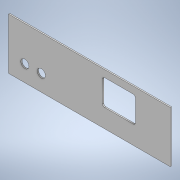
# Autodesk Inventor part: BackPanel
Saved by Autodesk Inventor 2021.4 (Build 254397000, 397)
## iProperties
Created: 2022-05-18
Part Number: BackPanel
Material: Generic
Document SubType Name: Modeling
Designer: LaborAdmin
Density: 1 g/cm^3
Appearance: Default
Author: LaborAdmin
Autodesk Inventor part; units mm, degrees
ref_plane "YZ Plane" through (0, 0, 0) normal (1, 0, 0) x (0, 1, 0)
ref_plane "XZ Plane" through (0, 0, 0) normal (0, 1, 0) x (-1, 0, 0)
ref_plane "XY Plane" through (0, 0, 0) normal (0, 0, 1) x (1, 0, 0)
sketch "Sketch1" plane through (0, 0, 0) normal (0, 0, 1) x (1, 0, 0)
  line L0 (-197, 62.5) -> (197, 62.5)
  line L1 (197, 62.5) -> (197, -62.5)
  line L2 (197, -62.5) -> (-197, -62.5)
  line L3 (-197, -62.5) -> (-197, 62.5)
  line L4 (-197, 62.5) -> (197, -62.5) construction
  line L5 (197, 62.5) -> (-197, -62.5) construction
  point P0 (0, 0)
  dimension "d0" = 394
  dimension "d1" = 125
  constraints: 12 end point, 2 midpoint, 2 parallel, 1 horizontal, 1 perpendicular
  measures "d0" distance of L1.end L2.end
  measures "d1" distance of L0.end L1.end
extrude "Extrusion1" add sketch "Sketch1" against normal blind 3
sketch "Sketch2" plane through (0, 0, 0) normal (0, 0, 1) x (1, 0, 0)
  circle A0 centre (-157, -22.5) radius 10
  circle A1 centre (-117, -22.5) radius 10
  line L0 (-197, -62.5) -> (197, -62.5) projected
  line L1 (-197, 62.5) -> (-197, -62.5) projected
  line L2 (37, 45.5) -> (107, 45.5)
  line L3 (112, 40.5) -> (112, -12.5)
  line L4 (107, -17.5) -> (37, -17.5)
  line L5 (32, -12.5) -> (32, 40.5)
  line L6 (197, 62.5) -> (-197, 62.5) projected
  line L7 (197, -62.5) -> (197, 62.5) projected
  arc A2 (37, 45.5) -> (32, 40.5) centre (37, 40.5) ccw
  arc A3 (112, 40.5) -> (107, 45.5) centre (107, 40.5) ccw
  arc A4 (107, -17.5) -> (112, -12.5) centre (107, -12.5) ccw
  arc A5 (32, -12.5) -> (37, -17.5) centre (37, -12.5) ccw
  point P0 (0, 0)
  point P1 (32, 45.5)
  point P2 (112, -17.5)
  point P3 (112, 45.5)
  point P4 (32, -17.5)
  dimension "d4" = 20
  dimension "USB" = 20
  dimension "d6" = 40
  dimension "d7" = 40
  dimension "d8" = 40
  dimension "d9" = 40
  dimension "d10" = 63
  dimension "d11" = 17
  dimension "d12" = 80
  dimension "d13" = 85
  dimension "d16" = 5
  constraints: 8 end point, 8 point on circle, 8 point on line, 8 tangent, 6 centre point, 3 equal radius, 2 parallel, 1 horizontal, 1 perpendicular
  measures "d4" diameter of A0
  measures "USB" diameter of A1
  measures "d6" distance from line of L0 A0.centre
  measures "d7" distance from line of L0 A1.centre
  measures "d8" distance from line of A0.centre L1
  measures "d9" distance of A1.centre A0.centre
  measures "d10" distance of point (32, -17.5) point (32, 45.5)
  measures "d11" distance between parallel lines of L6 L2
  measures "d12" distance between parallel lines of L5 L3
  measures "d13" distance between parallel lines of L7 L3
  measures "d16" radius of A2
extrude "Extrusion2" cut sketch "Sketch2" against normal blind 3 contours A0 | A1 | L2 A3 L3 A4 L4 A5 L5 A2
equation "\"d4\" = USB"
body "Solid1"
